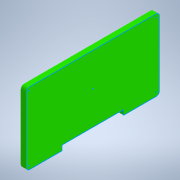
# Autodesk Inventor part: PCB
Saved by Autodesk Inventor 2021 (Build 250183000, 183)
## iProperties
Created: 2020-06-14
Part Number: PCB
Material: Generic
Document SubType Name: Modeling
Designer: drago
Density: 1 g/cm^3
Appearance: Default
Author: drago
Autodesk Inventor part; units mm, degrees
ref_plane "YZ Plane" through (0, 0, 0) normal (1, 0, 0) x (0, 1, 0)
ref_plane "XZ Plane" through (0, 0, 0) normal (0, 1, 0) x (-1, 0, 0)
ref_plane "XY Plane" through (0, 0, 0) normal (0, 0, 1) x (1, 0, 0)
sketch "Sketch1" plane through (0, 0, 0) normal (1, 0, 0) x (0, 1, 0)
  line L0 (10, 20) -> (-10, 20)
  line L1 (-10, 20) -> (-10, -20)
  line L2 (-10, -20) -> (10, -20)
  line L3 (10, -20) -> (10, 20)
  point P0 (0, 0)
  point P1 (-10, 20)
  dimension "d3" = 0
  dimension "d4" = 40
  dimension "d5" = 20
  dimension "d6" = 10
  dimension "d7" = 20
  constraints: 8 end point, 5 horizontal, 4 vertical, 2 parallel, 1 perpendicular, 16 other
  measures "d4" distance between parallel lines of L2 L0
  measures "d5" distance between parallel lines of L1 L3
  measures "d6" distance from line of point (0, 0) L3
  measures "d7" distance from line of point (0, 0) L0
extrude "Extrusion1" add sketch "Sketch1" along normal mid plane 1.6
sketch "Sketch3" plane through (0.8, 0, 0) normal (1, 0, 0) x (0, 0, -1)
  line L0 (-20, -10) -> (-9.25, -10)
  line L1 (-9.25, -10) -> (-9.25, -11.5)
  line L2 (-9.25, -11.5) -> (-20, -11.5)
  line L3 (-20, -11.5) -> (-20, -10)
  line L4 (-20, -10) -> (20, -10) projected
  line L5 (0, -15.8) -> (0, 14.3) projected
  line L6 (20, -10) -> (9.25, -10)
  line L7 (9.25, -10) -> (9.25, -11.5)
  line L8 (9.25, -11.5) -> (20, -11.5)
  line L9 (20, -11.5) -> (20, -10)
  line L10 (20, -10) -> (-20, -10)
  point P0 (0, 0)
  point P1 (9.25, -10)
  dimension "d10" = 1.5
  dimension "d11" = 9.25
  constraints: 18 end point, 5 symmetric about line, 2 parallel, 1 horizontal, 1 perpendicular
  measures "d10" distance between parallel lines of L4 L2
  measures "d11" distance between parallel lines of L5 L1
extrude "Extrusion2" add sketch "Sketch3" against normal up to surface (1.6 mm away)
fillet "Fillet1" radius 1 4 edges at (0, 10, 20) (0, -11.5, 20) (0, 10, -20) (0, -11.5, -20)
sketch "EXTENSION_MODULE_PSB_OUTLINE" plane through (-0.8, 0, 0) normal (-1, 0, 0) x (0, 0, 1)
  line L0 (20, 9) -> (20, -10.5) projected
  arc A0 (20, 9) -> (19, 10) centre (19, 9) ccw projected
  line L1 (19, 10) -> (-19, 10) projected
  arc A1 (-19, 10) -> (-20, 9) centre (-19, 9) ccw projected
  line L2 (-20, 9) -> (-20, -10.5) projected
  arc A2 (-20, -10.5) -> (-19, -11.5) centre (-19, -10.5) ccw projected
  line L3 (-9.25, -11.5) -> (-19, -11.5) projected
  arc A3 (19, -11.5) -> (20, -10.5) centre (19, -10.5) ccw projected
  line L4 (19, -11.5) -> (9.25, -11.5) projected
  line L5 (-9.25, -10) -> (-9.25, -11.5) projected
  line L6 (9.25, -11.5) -> (9.25, -10) projected
  line L7 (-9.25, -10) -> (9.25, -10) projected
  line L8 (-7.9375, -7.2568) -> (-7.9375, -10.762) projected
  line L9 (-7.3025, -10.762) -> (-7.3025, -7.2568) projected
  line L10 (7.3025, -7.2568) -> (7.3025, -10.762) projected
  line L11 (7.9375, -10.762) -> (7.9375, -7.2568) projected
  point P0 (0, 0)
sketch "ES_MODULE_OUTLINE" plane through (0.8, 0, 0) normal (1, 0, 0) x (0, 0, -1)
  arc A0 (19, -11.5) -> (20, -10.5) centre (19, -10.5) ccw projected
  line L0 (20, -10.5) -> (20, 9) projected
  arc A1 (20, 9) -> (19, 10) centre (19, 9) ccw projected
  line L1 (19, 10) -> (-19, 10) projected
  arc A2 (-19, 10) -> (-20, 9) centre (-19, 9) ccw projected
  line L2 (-20, 9) -> (-20, -10.5) projected
  arc A3 (-20, -10.5) -> (-19, -11.5) centre (-19, -10.5) ccw projected
  line L3 (-19, -11.5) -> (-9.25, -11.5) projected
  line L4 (-9.25, -11.5) -> (-9.25, -10) projected
  line L5 (-9.25, -10) -> (9.25, -10) projected
  line L6 (9.25, -10) -> (9.25, -11.5) projected
  line L7 (9.25, -11.5) -> (19, -11.5) projected
  point P0 (0, 0)
equation "\"d4\" = length"
equation "\"d5\" = height"
equation "\"d6\" = 0.5 * d5"
equation "\"d7\" = 0.5 * d4"
equation "\"d8\" = thickness"
equation "\"radious\" = 0"
equation "\"thickness\" = 1.6"
equation "\"length\" = 40"
equation "\"height\" = 20"
body "Solid1"
